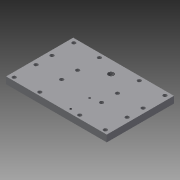
# Autodesk Inventor part: mobile plate
Saved by Autodesk Inventor 2015 SP1 (Build 190203100, 203)
## iProperties
Created: 2015-04-23
Part Number: mobile plate
Material: Generic
Document SubType Name: Modeling
Designer: ubik
Density: 1 g/cm^3
Appearance: Default
Author: ubik
Autodesk Inventor part; units mm, degrees
ref_plane "YZ Plane" through (0, 0, 0) normal (1, 0, 0) x (0, 1, 0)
ref_plane "XZ Plane" through (0, 0, 0) normal (0, 1, 0) x (-1, 0, 0)
ref_plane "XY Plane" through (0, 0, 0) normal (0, 0, 1) x (1, 0, 0)
sketch "Sketch1" plane through (0, 0, 0) normal (0, 0, 1) x (1, 0, 0)
  line L0 (0, 0) -> (120, 0)
  line L1 (120, 0) -> (120, 80)
  line L2 (120, 80) -> (0, 80)
  line L3 (0, 80) -> (0, 0)
  dimension "width" = 120
  dimension "height" = 80
  constraints: 8 end point, 2 parallel, 1 horizontal, 1 perpendicular
  measures "width" distance of L2.end L1.end
  measures "height" distance of L1.end L0.end
extrude "Extrusion1" add sketch "Sketch1" along normal blind 8
hole "Hole1" at (36.25, 75, 8) direction (0, 0, -1) diameter 4.5 end through all
pattern_linear "Rectangular Pattern1" count 2 spacing 30.5 along (-1, 0, 0) count 2 spacing 26 along (0, -1, 0) of "Hole1"
hole "Hole2" at (83.75, 75, 8) direction (0, 0, -1) diameter 4.5 end through all
pattern_linear "Rectangular Pattern2" count 2 spacing 30.5 along (1, 0, 0) count 2 spacing 26 along (0, -1, 0) of "Hole2"
pattern_linear "Rectangular Pattern3" count 2 spacing 45 along (0, -1, 0) of "Hole1", "Rectangular Pattern1", "Hole2", "Rectangular Pattern2"
hole "Hole3" at (60, 65, 8) direction (0, 0, -1) diameter 6.647 end through all thread size "M8x1.25" class "6H" standard "ANSI Metric M Profile"
hole "Hole4" at (72, 5, 8) direction (0, 0, -1) diameter 2.459 end through all thread size "M3x0.5" class "6H" standard "ANSI Metric M Profile"
hole "Hole5" at (72, 27.5, 8) direction (0, 0, -1) diameter 2.459 end through all thread size "M3x0.5" class "6H" standard "ANSI Metric M Profile"
equation "\"d37\" = 0.5 * width"
body "Solid1"
